Autodesk Inventor part; units mm, degrees
(part 3 of 4)
  arc A667 (-372.9607, 402.336) -> (-375.7104, 397.5735) centre (-372.9607, 399.161) ccw
  arc A668 (-368.5096, 385.1015) -> (-363.0104, 385.1015) centre (-365.76, 386.689) ccw
  line L673 (-355.8096, 397.5735) -> (-363.0104, 385.1015)
  line L674 (-372.9607, 402.336) -> (-358.5593, 402.336)
  arc A669 (-363.2031, 377.2287) -> (-368.7023, 377.2287) centre (-365.9527, 375.6412) ccw
  line L675 (-356.0023, 364.7567) -> (-363.2031, 377.2287)
  line L676 (-368.7023, 377.2287) -> (-375.9031, 364.7567)
  arc A670 (-375.9031, 364.7567) -> (-373.1534, 359.9942) centre (-373.1534, 363.1692) ccw
  line L677 (-373.1534, 359.9942) -> (-358.752, 359.9942)
  arc A671 (-358.752, 359.9942) -> (-356.0023, 364.7567) centre (-358.752, 363.1692) ccw
  line L678 (-314.1536, 58.9655) -> (-321.3544, 71.4375)
  arc A672 (-301.4536, 71.4375) -> (-304.2033, 76.2) centre (-304.2033, 73.025) ccw
  arc A673 (-318.6047, 76.2) -> (-321.3544, 71.4375) centre (-318.6047, 73.025) ccw
  arc A674 (-314.1536, 58.9655) -> (-308.6544, 58.9655) centre (-311.404, 60.553) ccw
  line L679 (-301.4536, 71.4375) -> (-308.6544, 58.9655)
  line L680 (-318.6047, 76.2) -> (-304.2033, 76.2)
  arc A675 (-308.8471, 51.0927) -> (-314.3463, 51.0927) centre (-311.5967, 49.5052) ccw
  line L681 (-301.6463, 38.6207) -> (-308.8471, 51.0927)
  line L682 (-314.3463, 51.0927) -> (-321.5471, 38.6207)
  arc A676 (-321.5471, 38.6207) -> (-318.7974, 33.8582) centre (-318.7974, 37.0332) ccw
  line L683 (-318.7974, 33.8582) -> (-304.396, 33.8582)
  arc A677 (-304.396, 33.8582) -> (-301.6463, 38.6207) centre (-304.396, 37.0332) ccw
  line L684 (-314.1536, 113.3215) -> (-321.3544, 125.7935)
  arc A678 (-301.4536, 125.7935) -> (-304.2033, 130.556) centre (-304.2033, 127.381) ccw
  arc A679 (-318.6047, 130.556) -> (-321.3544, 125.7935) centre (-318.6047, 127.381) ccw
  arc A680 (-314.1536, 113.3215) -> (-308.6544, 113.3215) centre (-311.404, 114.909) ccw
  line L685 (-301.4536, 125.7935) -> (-308.6544, 113.3215)
  line L686 (-318.6047, 130.556) -> (-304.2033, 130.556)
  arc A681 (-308.8471, 105.4487) -> (-314.3463, 105.4487) centre (-311.5967, 103.8612) ccw
  line L687 (-301.6463, 92.9767) -> (-308.8471, 105.4487)
  line L688 (-314.3463, 105.4487) -> (-321.5471, 92.9767)
  arc A682 (-321.5471, 92.9767) -> (-318.7974, 88.2142) centre (-318.7974, 91.3892) ccw
  line L689 (-318.7974, 88.2142) -> (-304.396, 88.2142)
  arc A683 (-304.396, 88.2142) -> (-301.6463, 92.9767) centre (-304.396, 91.3892) ccw
  line L690 (-314.1536, 167.6775) -> (-321.3544, 180.1495)
  arc A684 (-301.4536, 180.1495) -> (-304.2033, 184.912) centre (-304.2033, 181.737) ccw
  arc A685 (-318.6047, 184.912) -> (-321.3544, 180.1495) centre (-318.6047, 181.737) ccw
  arc A686 (-314.1536, 167.6775) -> (-308.6544, 167.6775) centre (-311.404, 169.265) ccw
  line L691 (-301.4536, 180.1495) -> (-308.6544, 167.6775)
  line L692 (-318.6047, 184.912) -> (-304.2033, 184.912)
  arc A687 (-308.8471, 159.8047) -> (-314.3463, 159.8047) centre (-311.5967, 158.2172) ccw
  line L693 (-301.6463, 147.3327) -> (-308.8471, 159.8047)
  line L694 (-314.3463, 159.8047) -> (-321.5471, 147.3327)
  arc A688 (-321.5471, 147.3327) -> (-318.7974, 142.5702) centre (-318.7974, 145.7452) ccw
  line L695 (-318.7974, 142.5702) -> (-304.396, 142.5702)
  arc A689 (-304.396, 142.5702) -> (-301.6463, 147.3327) centre (-304.396, 145.7452) ccw
  line L696 (-314.1536, 222.0335) -> (-321.3544, 234.5055)
  arc A690 (-301.4536, 234.5055) -> (-304.2033, 239.268) centre (-304.2033, 236.093) ccw
  arc A691 (-318.6047, 239.268) -> (-321.3544, 234.5055) centre (-318.6047, 236.093) ccw
  arc A692 (-314.1536, 222.0335) -> (-308.6544, 222.0335) centre (-311.404, 223.621) ccw
  line L697 (-301.4536, 234.5055) -> (-308.6544, 222.0335)
  line L698 (-318.6047, 239.268) -> (-304.2033, 239.268)
  arc A693 (-308.8471, 214.1607) -> (-314.3463, 214.1607) centre (-311.5967, 212.5732) ccw
  line L699 (-301.6463, 201.6887) -> (-308.8471, 214.1607)
  line L700 (-314.3463, 214.1607) -> (-321.5471, 201.6887)
  arc A694 (-321.5471, 201.6887) -> (-318.7974, 196.9262) centre (-318.7974, 200.1012) ccw
  line L701 (-318.7974, 196.9262) -> (-304.396, 196.9262)
  arc A695 (-304.396, 196.9262) -> (-301.6463, 201.6887) centre (-304.396, 200.1012) ccw
  line L702 (-314.1536, 276.3895) -> (-321.3544, 288.8615)
  arc A696 (-301.4536, 288.8615) -> (-304.2033, 293.624) centre (-304.2033, 290.449) ccw
  arc A697 (-318.6047, 293.624) -> (-321.3544, 288.8615) centre (-318.6047, 290.449) ccw
  arc A698 (-314.1536, 276.3895) -> (-308.6544, 276.3895) centre (-311.404, 277.977) ccw
  line L703 (-301.4536, 288.8615) -> (-308.6544, 276.3895)
  line L704 (-318.6047, 293.624) -> (-304.2033, 293.624)
  arc A699 (-308.8471, 268.5167) -> (-314.3463, 268.5167) centre (-311.5967, 266.9292) ccw
  line L705 (-301.6463, 256.0447) -> (-308.8471, 268.5167)
  line L706 (-314.3463, 268.5167) -> (-321.5471, 256.0447)
  arc A700 (-321.5471, 256.0447) -> (-318.7974, 251.2822) centre (-318.7974, 254.4572) ccw
  line L707 (-318.7974, 251.2822) -> (-304.396, 251.2822)
  arc A701 (-304.396, 251.2822) -> (-301.6463, 256.0447) centre (-304.396, 254.4572) ccw
  line L708 (-314.1536, 330.7455) -> (-321.3544, 343.2175)
  arc A702 (-301.4536, 343.2175) -> (-304.2033, 347.98) centre (-304.2033, 344.805) ccw
  arc A703 (-318.6047, 347.98) -> (-321.3544, 343.2175) centre (-318.6047, 344.805) ccw
  arc A704 (-314.1536, 330.7455) -> (-308.6544, 330.7455) centre (-311.404, 332.333) ccw
  line L709 (-301.4536, 343.2175) -> (-308.6544, 330.7455)
  line L710 (-318.6047, 347.98) -> (-304.2033, 347.98)
  arc A705 (-308.8471, 322.8727) -> (-314.3463, 322.8727) centre (-311.5967, 321.2852) ccw
  line L711 (-301.6463, 310.4007) -> (-308.8471, 322.8727)
  line L712 (-314.3463, 322.8727) -> (-321.5471, 310.4007)
  arc A706 (-321.5471, 310.4007) -> (-318.7974, 305.6382) centre (-318.7974, 308.8132) ccw
  line L713 (-318.7974, 305.6382) -> (-304.396, 305.6382)
  arc A707 (-304.396, 305.6382) -> (-301.6463, 310.4007) centre (-304.396, 308.8132) ccw
  line L714 (-314.1536, 385.1015) -> (-321.3544, 397.5735)
  arc A708 (-301.4536, 397.5735) -> (-304.2033, 402.336) centre (-304.2033, 399.161) ccw
  arc A709 (-318.6047, 402.336) -> (-321.3544, 397.5735) centre (-318.6047, 399.161) ccw
  arc A710 (-314.1536, 385.1015) -> (-308.6544, 385.1015) centre (-311.404, 386.689) ccw
  line L715 (-301.4536, 397.5735) -> (-308.6544, 385.1015)
  line L716 (-318.6047, 402.336) -> (-304.2033, 402.336)
  arc A711 (-308.8471, 377.2287) -> (-314.3463, 377.2287) centre (-311.5967, 375.6412) ccw
  line L717 (-301.6463, 364.7567) -> (-308.8471, 377.2287)
  line L718 (-314.3463, 377.2287) -> (-321.5471, 364.7567)
  arc A712 (-321.5471, 364.7567) -> (-318.7974, 359.9942) centre (-318.7974, 363.1692) ccw
  line L719 (-318.7974, 359.9942) -> (-304.396, 359.9942)
  arc A713 (-304.396, 359.9942) -> (-301.6463, 364.7567) centre (-304.396, 363.1692) ccw
  line L720 (-259.7976, 58.9655) -> (-266.9984, 71.4375)
  arc A714 (-247.0976, 71.4375) -> (-249.8473, 76.2) centre (-249.8473, 73.025) ccw
  arc A715 (-264.2487, 76.2) -> (-266.9984, 71.4375) centre (-264.2487, 73.025) ccw
  arc A716 (-259.7976, 58.9655) -> (-254.2984, 58.9655) centre (-257.048, 60.553) ccw
  line L721 (-247.0976, 71.4375) -> (-254.2984, 58.9655)
  line L722 (-264.2487, 76.2) -> (-249.8473, 76.2)
  arc A717 (-254.4911, 51.0927) -> (-259.9903, 51.0927) centre (-257.2407, 49.5052) ccw
  line L723 (-247.2903, 38.6207) -> (-254.4911, 51.0927)
  line L724 (-259.9903, 51.0927) -> (-267.1911, 38.6207)
  arc A718 (-267.1911, 38.6207) -> (-264.4414, 33.8582) centre (-264.4414, 37.0332) ccw
  line L725 (-264.4414, 33.8582) -> (-250.04, 33.8582)
  arc A719 (-250.04, 33.8582) -> (-247.2903, 38.6207) centre (-250.04, 37.0332) ccw
  line L726 (-259.7976, 113.3215) -> (-266.9984, 125.7935)
  arc A720 (-247.0976, 125.7935) -> (-249.8473, 130.556) centre (-249.8473, 127.381) ccw
  arc A721 (-264.2487, 130.556) -> (-266.9984, 125.7935) centre (-264.2487, 127.381) ccw
  arc A722 (-259.7976, 113.3215) -> (-254.2984, 113.3215) centre (-257.048, 114.909) ccw
  line L727 (-247.0976, 125.7935) -> (-254.2984, 113.3215)
  line L728 (-264.2487, 130.556) -> (-249.8473, 130.556)
  arc A723 (-254.4911, 105.4487) -> (-259.9903, 105.4487) centre (-257.2407, 103.8612) ccw
  line L729 (-247.2903, 92.9767) -> (-254.4911, 105.4487)
  line L730 (-259.9903, 105.4487) -> (-267.1911, 92.9767)
  arc A724 (-267.1911, 92.9767) -> (-264.4414, 88.2142) centre (-264.4414, 91.3892) ccw
  line L731 (-264.4414, 88.2142) -> (-250.04, 88.2142)
  arc A725 (-250.04, 88.2142) -> (-247.2903, 92.9767) centre (-250.04, 91.3892) ccw
  line L732 (-259.7976, 167.6775) -> (-266.9984, 180.1495)
  arc A726 (-247.0976, 180.1495) -> (-249.8473, 184.912) centre (-249.8473, 181.737) ccw
  arc A727 (-264.2487, 184.912) -> (-266.9984, 180.1495) centre (-264.2487, 181.737) ccw
  arc A728 (-259.7976, 167.6775) -> (-254.2984, 167.6775) centre (-257.048, 169.265) ccw
  line L733 (-247.0976, 180.1495) -> (-254.2984, 167.6775)
  line L734 (-264.2487, 184.912) -> (-249.8473, 184.912)
  arc A729 (-254.4911, 159.8047) -> (-259.9903, 159.8047) centre (-257.2407, 158.2172) ccw
  line L735 (-247.2903, 147.3327) -> (-254.4911, 159.8047)
  line L736 (-259.9903, 159.8047) -> (-267.1911, 147.3327)
  arc A730 (-267.1911, 147.3327) -> (-264.4414, 142.5702) centre (-264.4414, 145.7452) ccw
  line L737 (-264.4414, 142.5702) -> (-250.04, 142.5702)
  arc A731 (-250.04, 142.5702) -> (-247.2903, 147.3327) centre (-250.04, 145.7452) ccw
  line L738 (-259.7976, 222.0335) -> (-266.9984, 234.5055)
  arc A732 (-247.0976, 234.5055) -> (-249.8473, 239.268) centre (-249.8473, 236.093) ccw
  arc A733 (-264.2487, 239.268) -> (-266.9984, 234.5055) centre (-264.2487, 236.093) ccw
  arc A734 (-259.7976, 222.0335) -> (-254.2984, 222.0335) centre (-257.048, 223.621) ccw
  line L739 (-247.0976, 234.5055) -> (-254.2984, 222.0335)
  line L740 (-264.2487, 239.268) -> (-249.8473, 239.268)
  arc A735 (-254.4911, 214.1607) -> (-259.9903, 214.1607) centre (-257.2407, 212.5732) ccw
  line L741 (-247.2903, 201.6887) -> (-254.4911, 214.1607)
  line L742 (-259.9903, 214.1607) -> (-267.1911, 201.6887)
  arc A736 (-267.1911, 201.6887) -> (-264.4414, 196.9262) centre (-264.4414, 200.1012) ccw
  line L743 (-264.4414, 196.9262) -> (-250.04, 196.9262)
  arc A737 (-250.04, 196.9262) -> (-247.2903, 201.6887) centre (-250.04, 200.1012) ccw
  line L744 (-259.7976, 276.3895) -> (-266.9984, 288.8615)
  arc A738 (-247.0976, 288.8615) -> (-249.8473, 293.624) centre (-249.8473, 290.449) ccw
  arc A739 (-264.2487, 293.624) -> (-266.9984, 288.8615) centre (-264.2487, 290.449) ccw
  arc A740 (-259.7976, 276.3895) -> (-254.2984, 276.3895) centre (-257.048, 277.977) ccw
  line L745 (-247.0976, 288.8615) -> (-254.2984, 276.3895)
  line L746 (-264.2487, 293.624) -> (-249.8473, 293.624)
  arc A741 (-254.4911, 268.5167) -> (-259.9903, 268.5167) centre (-257.2407, 266.9292) ccw
  line L747 (-247.2903, 256.0447) -> (-254.4911, 268.5167)
  line L748 (-259.9903, 268.5167) -> (-267.1911, 256.0447)
  arc A742 (-267.1911, 256.0447) -> (-264.4414, 251.2822) centre (-264.4414, 254.4572) ccw
  line L749 (-264.4414, 251.2822) -> (-250.04, 251.2822)
  arc A743 (-250.04, 251.2822) -> (-247.2903, 256.0447) centre (-250.04, 254.4572) ccw
  line L750 (-259.7976, 330.7455) -> (-266.9984, 343.2175)
  arc A744 (-247.0976, 343.2175) -> (-249.8473, 347.98) centre (-249.8473, 344.805) ccw
  arc A745 (-264.2487, 347.98) -> (-266.9984, 343.2175) centre (-264.2487, 344.805) ccw
  arc A746 (-259.7976, 330.7455) -> (-254.2984, 330.7455) centre (-257.048, 332.333) ccw
  line L751 (-247.0976, 343.2175) -> (-254.2984, 330.7455)
  line L752 (-264.2487, 347.98) -> (-249.8473, 347.98)
  arc A747 (-254.4911, 322.8727) -> (-259.9903, 322.8727) centre (-257.2407, 321.2852) ccw
  line L753 (-247.2903, 310.4007) -> (-254.4911, 322.8727)
  line L754 (-259.9903, 322.8727) -> (-267.1911, 310.4007)
  arc A748 (-267.1911, 310.4007) -> (-264.4414, 305.6382) centre (-264.4414, 308.8132) ccw
  line L755 (-264.4414, 305.6382) -> (-250.04, 305.6382)
  arc A749 (-250.04, 305.6382) -> (-247.2903, 310.4007) centre (-250.04, 308.8132) ccw
  line L756 (-259.7976, 385.1015) -> (-266.9984, 397.5735)
  arc A750 (-247.0976, 397.5735) -> (-249.8473, 402.336) centre (-249.8473, 399.161) ccw
  arc A751 (-264.2487, 402.336) -> (-266.9984, 397.5735) centre (-264.2487, 399.161) ccw
  arc A752 (-259.7976, 385.1015) -> (-254.2984, 385.1015) centre (-257.048, 386.689) ccw
  line L757 (-247.0976, 397.5735) -> (-254.2984, 385.1015)
  line L758 (-264.2487, 402.336) -> (-249.8473, 402.336)
  arc A753 (-254.4911, 377.2287) -> (-259.9903, 377.2287) centre (-257.2407, 375.6412) ccw
  line L759 (-247.2903, 364.7567) -> (-254.4911, 377.2287)
  line L760 (-259.9903, 377.2287) -> (-267.1911, 364.7567)
  arc A754 (-267.1911, 364.7567) -> (-264.4414, 359.9942) centre (-264.4414, 363.1692) ccw
  line L761 (-264.4414, 359.9942) -> (-250.04, 359.9942)
  arc A755 (-250.04, 359.9942) -> (-247.2903, 364.7567) centre (-250.04, 363.1692) ccw
  line L762 (-205.4416, 58.9655) -> (-212.6424, 71.4375)
  arc A756 (-192.7416, 71.4375) -> (-195.4913, 76.2) centre (-195.4913, 73.025) ccw
  arc A757 (-209.8927, 76.2) -> (-212.6424, 71.4375) centre (-209.8927, 73.025) ccw
  arc A758 (-205.4416, 58.9655) -> (-199.9424, 58.9655) centre (-202.692, 60.553) ccw
  line L763 (-192.7416, 71.4375) -> (-199.9424, 58.9655)
  line L764 (-209.8927, 76.2) -> (-195.4913, 76.2)
  arc A759 (-200.1351, 51.0927) -> (-205.6343, 51.0927) centre (-202.8847, 49.5052) ccw
  line L765 (-192.9343, 38.6207) -> (-200.1351, 51.0927)
  line L766 (-205.6343, 51.0927) -> (-212.8351, 38.6207)
  arc A760 (-212.8351, 38.6207) -> (-210.0854, 33.8582) centre (-210.0854, 37.0332) ccw
  line L767 (-210.0854, 33.8582) -> (-195.684, 33.8582)
  arc A761 (-195.684, 33.8582) -> (-192.9343, 38.6207) centre (-195.684, 37.0332) ccw
  line L768 (-205.4416, 113.3215) -> (-212.6424, 125.7935)
  arc A762 (-192.7416, 125.7935) -> (-195.4913, 130.556) centre (-195.4913, 127.381) ccw
  arc A763 (-209.8927, 130.556) -> (-212.6424, 125.7935) centre (-209.8927, 127.381) ccw
  arc A764 (-205.4416, 113.3215) -> (-199.9424, 113.3215) centre (-202.692, 114.909) ccw
  line L769 (-192.7416, 125.7935) -> (-199.9424, 113.3215)
  line L770 (-209.8927, 130.556) -> (-195.4913, 130.556)
  arc A765 (-200.1351, 105.4487) -> (-205.6343, 105.4487) centre (-202.8847, 103.8612) ccw
  line L771 (-192.9343, 92.9767) -> (-200.1351, 105.4487)
  line L772 (-205.6343, 105.4487) -> (-212.8351, 92.9767)
  arc A766 (-212.8351, 92.9767) -> (-210.0854, 88.2142) centre (-210.0854, 91.3892) ccw
  line L773 (-210.0854, 88.2142) -> (-195.684, 88.2142)
  arc A767 (-195.684, 88.2142) -> (-192.9343, 92.9767) centre (-195.684, 91.3892) ccw
  line L774 (-205.4416, 167.6775) -> (-212.6424, 180.1495)
  arc A768 (-192.7416, 180.1495) -> (-195.4913, 184.912) centre (-195.4913, 181.737) ccw
  arc A769 (-209.8927, 184.912) -> (-212.6424, 180.1495) centre (-209.8927, 181.737) ccw
  arc A770 (-205.4416, 167.6775) -> (-199.9424, 167.6775) centre (-202.692, 169.265) ccw
  line L775 (-192.7416, 180.1495) -> (-199.9424, 167.6775)
  line L776 (-209.8927, 184.912) -> (-195.4913, 184.912)
  arc A771 (-200.1351, 159.8047) -> (-205.6343, 159.8047) centre (-202.8847, 158.2172) ccw
  line L777 (-192.9343, 147.3327) -> (-200.1351, 159.8047)
  line L778 (-205.6343, 159.8047) -> (-212.8351, 147.3327)
  arc A772 (-212.8351, 147.3327) -> (-210.0854, 142.5702) centre (-210.0854, 145.7452) ccw
  line L779 (-210.0854, 142.5702) -> (-195.684, 142.5702)
  arc A773 (-195.684, 142.5702) -> (-192.9343, 147.3327) centre (-195.684, 145.7452) ccw
  line L780 (-205.4416, 222.0335) -> (-212.6424, 234.5055)
  arc A774 (-192.7416, 234.5055) -> (-195.4913, 239.268) centre (-195.4913, 236.093) ccw
  arc A775 (-209.8927, 239.268) -> (-212.6424, 234.5055) centre (-209.8927, 236.093) ccw
  arc A776 (-205.4416, 222.0335) -> (-199.9424, 222.0335) centre (-202.692, 223.621) ccw
  line L781 (-192.7416, 234.5055) -> (-199.9424, 222.0335)
  line L782 (-209.8927, 239.268) -> (-195.4913, 239.268)
  arc A777 (-200.1351, 214.1607) -> (-205.6343, 214.1607) centre (-202.8847, 212.5732) ccw
  line L783 (-192.9343, 201.6887) -> (-200.1351, 214.1607)
  line L784 (-205.6343, 214.1607) -> (-212.8351, 201.6887)
  arc A778 (-212.8351, 201.6887) -> (-210.0854, 196.9262) centre (-210.0854, 200.1012) ccw
  line L785 (-210.0854, 196.9262) -> (-195.684, 196.9262)
  arc A779 (-195.684, 196.9262) -> (-192.9343, 201.6887) centre (-195.684, 200.1012) ccw
  line L786 (-205.4416, 276.3895) -> (-212.6424, 288.8615)
  arc A780 (-192.7416, 288.8615) -> (-195.4913, 293.624) centre (-195.4913, 290.449) ccw
  arc A781 (-209.8927, 293.624) -> (-212.6424, 288.8615) centre (-209.8927, 290.449) ccw
  arc A782 (-205.4416, 276.3895) -> (-199.9424, 276.3895) centre (-202.692, 277.977) ccw
  line L787 (-192.7416, 288.8615) -> (-199.9424, 276.3895)
  line L788 (-209.8927, 293.624) -> (-195.4913, 293.624)
  arc A783 (-200.1351, 268.5167) -> (-205.6343, 268.5167) centre (-202.8847, 266.9292) ccw
  line L789 (-192.9343, 256.0447) -> (-200.1351, 268.5167)
  line L790 (-205.6343, 268.5167) -> (-212.8351, 256.0447)
  arc A784 (-212.8351, 256.0447) -> (-210.0854, 251.2822) centre (-210.0854, 254.4572) ccw
  line L791 (-210.0854, 251.2822) -> (-195.684, 251.2822)
  arc A785 (-195.684, 251.2822) -> (-192.9343, 256.0447) centre (-195.684, 254.4572) ccw
  line L792 (-205.4416, 330.7455) -> (-212.6424, 343.2175)
  arc A786 (-192.7416, 343.2175) -> (-195.4913, 347.98) centre (-195.4913, 344.805) ccw
  arc A787 (-209.8927, 347.98) -> (-212.6424, 343.2175) centre (-209.8927, 344.805) ccw
  arc A788 (-205.4416, 330.7455) -> (-199.9424, 330.7455) centre (-202.692, 332.333) ccw
  line L793 (-192.7416, 343.2175) -> (-199.9424, 330.7455)
  line L794 (-209.8927, 347.98) -> (-195.4913, 347.98)
  arc A789 (-200.1351, 322.8727) -> (-205.6343, 322.8727) centre (-202.8847, 321.2852) ccw
  line L795 (-192.9343, 310.4007) -> (-200.1351, 322.8727)
  line L796 (-205.6343, 322.8727) -> (-212.8351, 310.4007)
  arc A790 (-212.8351, 310.4007) -> (-210.0854, 305.6382) centre (-210.0854, 308.8132) ccw
  line L797 (-210.0854, 305.6382) -> (-195.684, 305.6382)
  arc A791 (-195.684, 305.6382) -> (-192.9343, 310.4007) centre (-195.684, 308.8132) ccw
  line L798 (-205.4416, 385.1015) -> (-212.6424, 397.5735)
  arc A792 (-192.7416, 397.5735) -> (-195.4913, 402.336) centre (-195.4913, 399.161) ccw
  arc A793 (-209.8927, 402.336) -> (-212.6424, 397.5735) centre (-209.8927, 399.161) ccw
  arc A794 (-205.4416, 385.1015) -> (-199.9424, 385.1015) centre (-202.692, 386.689) ccw
  line L799 (-192.7416, 397.5735) -> (-199.9424, 385.1015)
  line L800 (-209.8927, 402.336) -> (-195.4913, 402.336)
  arc A795 (-200.1351, 377.2287) -> (-205.6343, 377.2287) centre (-202.8847, 375.6412) ccw
  line L801 (-192.9343, 364.7567) -> (-200.1351, 377.2287)
  line L802 (-205.6343, 377.2287) -> (-212.8351, 364.7567)
  arc A796 (-212.8351, 364.7567) -> (-210.0854, 359.9942) centre (-210.0854, 363.1692) ccw
  line L803 (-210.0854, 359.9942) -> (-195.684, 359.9942)
  arc A797 (-195.684, 359.9942) -> (-192.9343, 364.7567) centre (-195.684, 363.1692) ccw
  line L804 (-151.0856, 58.9655) -> (-158.2864, 71.4375)
  arc A798 (-138.3856, 71.4375) -> (-141.1353, 76.2) centre (-141.1353, 73.025) ccw
  arc A799 (-155.5367, 76.2) -> (-158.2864, 71.4375) centre (-155.5367, 73.025) ccw
  arc A800 (-151.0856, 58.9655) -> (-145.5864, 58.9655) centre (-148.336, 60.553) ccw
  line L805 (-138.3856, 71.4375) -> (-145.5864, 58.9655)
  line L806 (-155.5367, 76.2) -> (-141.1353, 76.2)
  arc A801 (-145.7791, 51.0927) -> (-151.2783, 51.0927) centre (-148.5287, 49.5052) ccw
  line L807 (-138.5783, 38.6207) -> (-145.7791, 51.0927)
  line L808 (-151.2783, 51.0927) -> (-158.4791, 38.6207)
  arc A802 (-158.4791, 38.6207) -> (-155.7294, 33.8582) centre (-155.7294, 37.0332) ccw
  line L809 (-155.7294, 33.8582) -> (-141.328, 33.8582)
  arc A803 (-141.328, 33.8582) -> (-138.5783, 38.6207) centre (-141.328, 37.0332) ccw
  line L810 (-151.0856, 113.3215) -> (-158.2864, 125.7935)
  arc A804 (-138.3856, 125.7935) -> (-141.1353, 130.556) centre (-141.1353, 127.381) ccw
  arc A805 (-155.5367, 130.556) -> (-158.2864, 125.7935) centre (-155.5367, 127.381) ccw
  arc A806 (-151.0856, 113.3215) -> (-145.5864, 113.3215) centre (-148.336, 114.909) ccw
  line L811 (-138.3856, 125.7935) -> (-145.5864, 113.3215)
  line L812 (-155.5367, 130.556) -> (-141.1353, 130.556)
  arc A807 (-145.7791, 105.4487) -> (-151.2783, 105.4487) centre (-148.5287, 103.8612) ccw
  line L813 (-138.5783, 92.9767) -> (-145.7791, 105.4487)
  line L814 (-151.2783, 105.4487) -> (-158.4791, 92.9767)
  arc A808 (-158.4791, 92.9767) -> (-155.7294, 88.2142) centre (-155.7294, 91.3892) ccw
  line L815 (-155.7294, 88.2142) -> (-141.328, 88.2142)
  arc A809 (-141.328, 88.2142) -> (-138.5783, 92.9767) centre (-141.328, 91.3892) ccw
  line L816 (-151.0856, 167.6775) -> (-158.2864, 180.1495)
  arc A810 (-138.3856, 180.1495) -> (-141.1353, 184.912) centre (-141.1353, 181.737) ccw
  arc A811 (-155.5367, 184.912) -> (-158.2864, 180.1495) centre (-155.5367, 181.737) ccw
  arc A812 (-151.0856, 167.6775) -> (-145.5864, 167.6775) centre (-148.336, 169.265) ccw
  line L817 (-138.3856, 180.1495) -> (-145.5864, 167.6775)
  line L818 (-155.5367, 184.912) -> (-141.1353, 184.912)
  arc A813 (-145.7791, 159.8047) -> (-151.2783, 159.8047) centre (-148.5287, 158.2172) ccw
  line L819 (-138.5783, 147.3327) -> (-145.7791, 159.8047)
  line L820 (-151.2783, 159.8047) -> (-158.4791, 147.3327)
  arc A814 (-158.4791, 147.3327) -> (-155.7294, 142.5702) centre (-155.7294, 145.7452) ccw
  line L821 (-155.7294, 142.5702) -> (-141.328, 142.5702)
  arc A815 (-141.328, 142.5702) -> (-138.5783, 147.3327) centre (-141.328, 145.7452) ccw
  line L822 (-151.0856, 222.0335) -> (-158.2864, 234.5055)
  arc A816 (-138.3856, 234.5055) -> (-141.1353, 239.268) centre (-141.1353, 236.093) ccw
  arc A817 (-155.5367, 239.268) -> (-158.2864, 234.5055) centre (-155.5367, 236.093) ccw
  arc A818 (-151.0856, 222.0335) -> (-145.5864, 222.0335) centre (-148.336, 223.621) ccw
  line L823 (-138.3856, 234.5055) -> (-145.5864, 222.0335)
  line L824 (-155.5367, 239.268) -> (-141.1353, 239.268)
  arc A819 (-145.7791, 214.1607) -> (-151.2783, 214.1607) centre (-148.5287, 212.5732) ccw
  line L825 (-138.5783, 201.6887) -> (-145.7791, 214.1607)
  line L826 (-151.2783, 214.1607) -> (-158.4791, 201.6887)
  arc A820 (-158.4791, 201.6887) -> (-155.7294, 196.9262) centre (-155.7294, 200.1012) ccw
  line L827 (-155.7294, 196.9262) -> (-141.328, 196.9262)
  arc A821 (-141.328, 196.9262) -> (-138.5783, 201.6887) centre (-141.328, 200.1012) ccw
  line L828 (-151.0856, 276.3895) -> (-158.2864, 288.8615)
  arc A822 (-138.3856, 288.8615) -> (-141.1353, 293.624) centre (-141.1353, 290.449) ccw
  arc A823 (-155.5367, 293.624) -> (-158.2864, 288.8615) centre (-155.5367, 290.449) ccw
  arc A824 (-151.0856, 276.3895) -> (-145.5864, 276.3895) centre (-148.336, 277.977) ccw
  line L829 (-138.3856, 288.8615) -> (-145.5864, 276.3895)
  line L830 (-155.5367, 293.624) -> (-141.1353, 293.624)
  arc A825 (-145.7791, 268.5167) -> (-151.2783, 268.5167) centre (-148.5287, 266.9292) ccw
  line L831 (-138.5783, 256.0447) -> (-145.7791, 268.5167)
  line L832 (-151.2783, 268.5167) -> (-158.4791, 256.0447)
  arc A826 (-158.4791, 256.0447) -> (-155.7294, 251.2822) centre (-155.7294, 254.4572) ccw
  line L833 (-155.7294, 251.2822) -> (-141.328, 251.2822)
  arc A827 (-141.328, 251.2822) -> (-138.5783, 256.0447) centre (-141.328, 254.4572) ccw
  line L834 (-151.0856, 330.7455) -> (-158.2864, 343.2175)
  arc A828 (-138.3856, 343.2175) -> (-141.1353, 347.98) centre (-141.1353, 344.805) ccw
  arc A829 (-155.5367, 347.98) -> (-158.2864, 343.2175) centre (-155.5367, 344.805) ccw
  arc A830 (-151.0856, 330.7455) -> (-145.5864, 330.7455) centre (-148.336, 332.333) ccw
  line L835 (-138.3856, 343.2175) -> (-145.5864, 330.7455)
  line L836 (-155.5367, 347.98) -> (-141.1353, 347.98)
  arc A831 (-145.7791, 322.8727) -> (-151.2783, 322.8727) centre (-148.5287, 321.2852) ccw
  line L837 (-138.5783, 310.4007) -> (-145.7791, 322.8727)
  line L838 (-151.2783, 322.8727) -> (-158.4791, 310.4007)
  arc A832 (-158.4791, 310.4007) -> (-155.7294, 305.6382) centre (-155.7294, 308.8132) ccw
  line L839 (-155.7294, 305.6382) -> (-141.328, 305.6382)
  arc A833 (-141.328, 305.6382) -> (-138.5783, 310.4007) centre (-141.328, 308.8132) ccw
  line L840 (-151.0856, 385.1015) -> (-158.2864, 397.5735)
  arc A834 (-138.3856, 397.5735) -> (-141.1353, 402.336) centre (-141.1353, 399.161) ccw
  arc A835 (-155.5367, 402.336) -> (-158.2864, 397.5735) centre (-155.5367, 399.161) ccw
  arc A836 (-151.0856, 385.1015) -> (-145.5864, 385.1015) centre (-148.336, 386.689) ccw
  line L841 (-138.3856, 397.5735) -> (-145.5864, 385.1015)
  line L842 (-155.5367, 402.336) -> (-141.1353, 402.336)
  arc A837 (-145.7791, 377.2287) -> (-151.2783, 377.2287) centre (-148.5287, 375.6412) ccw
  line L843 (-138.5783, 364.7567) -> (-145.7791, 377.2287)
  line L844 (-151.2783, 377.2287) -> (-158.4791, 364.7567)
  arc A838 (-158.4791, 364.7567) -> (-155.7294, 359.9942) centre (-155.7294, 363.1692) ccw
  line L845 (-155.7294, 359.9942) -> (-141.328, 359.9942)
  arc A839 (-141.328, 359.9942) -> (-138.5783, 364.7567) centre (-141.328, 363.1692) ccw
  line L846 (-96.7296, 58.9655) -> (-103.9304, 71.4375)
  arc A840 (-84.0296, 71.4375) -> (-86.7793, 76.2) centre (-86.7793, 73.025) ccw
  arc A841 (-101.1807, 76.2) -> (-103.9304, 71.4375) centre (-101.1807, 73.025) ccw
  arc A842 (-96.7296, 58.9655) -> (-91.2304, 58.9655) centre (-93.98, 60.553) ccw
  line L847 (-84.0296, 71.4375) -> (-91.2304, 58.9655)
  line L848 (-101.1807, 76.2) -> (-86.7793, 76.2)
  arc A843 (-91.4231, 51.0927) -> (-96.9223, 51.0927) centre (-94.1727, 49.5052) ccw
  line L849 (-84.2223, 38.6207) -> (-91.4231, 51.0927)
  line L850 (-96.9223, 51.0927) -> (-104.1231, 38.6207)
  arc A844 (-104.1231, 38.6207) -> (-101.3734, 33.8582) centre (-101.3734, 37.0332) ccw
  line L851 (-101.3734, 33.8582) -> (-86.972, 33.8582)
  arc A845 (-86.972, 33.8582) -> (-84.2223, 38.6207) centre (-86.972, 37.0332) ccw
  line L852 (-96.7296, 113.3215) -> (-103.9304, 125.7935)
  arc A846 (-84.0296, 125.7935) -> (-86.7793, 130.556) centre (-86.7793, 127.381) ccw
  arc A847 (-101.1807, 130.556) -> (-103.9304, 125.7935) centre (-101.1807, 127.381) ccw
  arc A848 (-96.7296, 113.3215) -> (-91.2304, 113.3215) centre (-93.98, 114.909) ccw
  line L853 (-84.0296, 125.7935) -> (-91.2304, 113.3215)
  line L854 (-101.1807, 130.556) -> (-86.7793, 130.556)
  arc A849 (-91.4231, 105.4487) -> (-96.9223, 105.4487) centre (-94.1727, 103.8612) ccw
  line L855 (-84.2223, 92.9767) -> (-91.4231, 105.4487)
  line L856 (-96.9223, 105.4487) -> (-104.1231, 92.9767)
  arc A850 (-104.1231, 92.9767) -> (-101.3734, 88.2142) centre (-101.3734, 91.3892) ccw
  line L857 (-101.3734, 88.2142) -> (-86.972, 88.2142)
  arc A851 (-86.972, 88.2142) -> (-84.2223, 92.9767) centre (-86.972, 91.3892) ccw
  line L858 (-96.7296, 167.6775) -> (-103.9304, 180.1495)
  arc A852 (-84.0296, 180.1495) -> (-86.7793, 184.912) centre (-86.7793, 181.737) ccw
  arc A853 (-101.1807, 184.912) -> (-103.9304, 180.1495) centre (-101.1807, 181.737) ccw
  arc A854 (-96.7296, 167.6775) -> (-91.2304, 167.6775) centre (-93.98, 169.265) ccw
  line L859 (-84.0296, 180.1495) -> (-91.2304, 167.6775)
  line L860 (-101.1807, 184.912) -> (-86.7793, 184.912)
  arc A855 (-91.4231, 159.8047) -> (-96.9223, 159.8047) centre (-94.1727, 158.2172) ccw
  line L861 (-84.2223, 147.3327) -> (-91.4231, 159.8047)
  line L862 (-96.9223, 159.8047) -> (-104.1231, 147.3327)
  arc A856 (-104.1231, 147.3327) -> (-101.3734, 142.5702) centre (-101.3734, 145.7452) ccw
  line L863 (-101.3734, 142.5702) -> (-86.972, 142.5702)
  arc A857 (-86.972, 142.5702) -> (-84.2223, 147.3327) centre (-86.972, 145.7452) ccw
  line L864 (-96.7296, 222.0335) -> (-103.9304, 234.5055)
  arc A858 (-84.0296, 234.5055) -> (-86.7793, 239.268) centre (-86.7793, 236.093) ccw
  arc A859 (-101.1807, 239.268) -> (-103.9304, 234.5055) centre (-101.1807, 236.093) ccw
  arc A860 (-96.7296, 222.0335) -> (-91.2304, 222.0335) centre (-93.98, 223.621) ccw
  line L865 (-84.0296, 234.5055) -> (-91.2304, 222.0335)
  line L866 (-101.1807, 239.268) -> (-86.7793, 239.268)
  arc A861 (-91.4231, 214.1607) -> (-96.9223, 214.1607) centre (-94.1727, 212.5732) ccw
  line L867 (-84.2223, 201.6887) -> (-91.4231, 214.1607)
  line L868 (-96.9223, 214.1607) -> (-104.1231, 201.6887)
  arc A862 (-104.1231, 201.6887) -> (-101.3734, 196.9262) centre (-101.3734, 200.1012) ccw
  line L869 (-101.3734, 196.9262) -> (-86.972, 196.9262)
  arc A863 (-86.972, 196.9262) -> (-84.2223, 201.6887) centre (-86.972, 200.1012) ccw
  line L870 (-96.7296, 276.3895) -> (-103.9304, 288.8615)
  arc A864 (-84.0296, 288.8615) -> (-86.7793, 293.624) centre (-86.7793, 290.449) ccw
  arc A865 (-101.1807, 293.624) -> (-103.9304, 288.8615) centre (-101.1807, 290.449) ccw
  arc A866 (-96.7296, 276.3895) -> (-91.2304, 276.3895) centre (-93.98, 277.977) ccw
  line L871 (-84.0296, 288.8615) -> (-91.2304, 276.3895)
  line L872 (-101.1807, 293.624) -> (-86.7793, 293.624)
  arc A867 (-91.4231, 268.5167) -> (-96.9223, 268.5167) centre (-94.1727, 266.9292) ccw
  line L873 (-84.2223, 256.0447) -> (-91.4231, 268.5167)
  line L874 (-96.9223, 268.5167) -> (-104.1231, 256.0447)
  arc A868 (-104.1231, 256.0447) -> (-101.3734, 251.2822) centre (-101.3734, 254.4572) ccw
  line L875 (-101.3734, 251.2822) -> (-86.972, 251.2822)
  arc A869 (-86.972, 251.2822) -> (-84.2223, 256.0447) centre (-86.972, 254.4572) ccw
  line L876 (-96.7296, 330.7455) -> (-103.9304, 343.2175)
  arc A870 (-84.0296, 343.2175) -> (-86.7793, 347.98) centre (-86.7793, 344.805) ccw
  arc A871 (-101.1807, 347.98) -> (-103.9304, 343.2175) centre (-101.1807, 344.805) ccw
  arc A872 (-96.7296, 330.7455) -> (-91.2304, 330.7455) centre (-93.98, 332.333) ccw
  line L877 (-84.0296, 343.2175) -> (-91.2304, 330.7455)
  line L878 (-101.1807, 347.98) -> (-86.7793, 347.98)
  arc A873 (-91.4231, 322.8727) -> (-96.9223, 322.8727) centre (-94.1727, 321.2852) ccw
  line L879 (-84.2223, 310.4007) -> (-91.4231, 322.8727)
  line L880 (-96.9223, 322.8727) -> (-104.1231, 310.4007)
  arc A874 (-104.1231, 310.4007) -> (-101.3734, 305.6382) centre (-101.3734, 308.8132) ccw
  line L881 (-101.3734, 305.6382) -> (-86.972, 305.6382)
  arc A875 (-86.972, 305.6382) -> (-84.2223, 310.4007) centre (-86.972, 308.8132) ccw
  line L882 (-96.7296, 385.1015) -> (-103.9304, 397.5735)
  arc A876 (-84.0296, 397.5735) -> (-86.7793, 402.336) centre (-86.7793, 399.161) ccw
  arc A877 (-101.1807, 402.336) -> (-103.9304, 397.5735) centre (-101.1807, 399.161) ccw
  arc A878 (-96.7296, 385.1015) -> (-91.2304, 385.1015) centre (-93.98, 386.689) ccw
  line L883 (-84.0296, 397.5735) -> (-91.2304, 385.1015)
  line L884 (-101.1807, 402.336) -> (-86.7793, 402.336)
  arc A879 (-91.4231, 377.2287) -> (-96.9223, 377.2287) centre (-94.1727, 375.6412) ccw
  line L885 (-84.2223, 364.7567) -> (-91.4231, 377.2287)
  line L886 (-96.9223, 377.2287) -> (-104.1231, 364.7567)
  arc A880 (-104.1231, 364.7567) -> (-101.3734, 359.9942) centre (-101.3734, 363.1692) ccw
  line L887 (-101.3734, 359.9942) -> (-86.972, 359.9942)
  arc A881 (-86.972, 359.9942) -> (-84.2223, 364.7567) centre (-86.972, 363.1692) ccw
  line L888 (-42.3736, 58.9655) -> (-49.5744, 71.4375)
  arc A882 (-29.6736, 71.4375) -> (-32.4233, 76.2) centre (-32.4233, 73.025) ccw
  arc A883 (-46.8247, 76.2) -> (-49.5744, 71.4375) centre (-46.8247, 73.025) ccw
  arc A884 (-42.3736, 58.9655) -> (-36.8744, 58.9655) centre (-39.624, 60.553) ccw
  line L889 (-29.6736, 71.4375) -> (-36.8744, 58.9655)
  line L890 (-46.8247, 76.2) -> (-32.4233, 76.2)
  arc A885 (-37.0671, 51.0927) -> (-42.5663, 51.0927) centre (-39.8167, 49.5052) ccw
  line L891 (-29.8663, 38.6207) -> (-37.0671, 51.0927)
  line L892 (-42.5663, 51.0927) -> (-49.7671, 38.6207)
  arc A886 (-49.7671, 38.6207) -> (-47.0174, 33.8582) centre (-47.0174, 37.0332) ccw
  line L893 (-47.0174, 33.8582) -> (-32.616, 33.8582)
  arc A887 (-32.616, 33.8582) -> (-29.8663, 38.6207) centre (-32.616, 37.0332) ccw
  line L894 (-42.3736, 113.3215) -> (-49.5744, 125.7935)
  arc A888 (-29.6736, 125.7935) -> (-32.4233, 130.556) centre (-32.4233, 127.381) ccw
  arc A889 (-46.8247, 130.556) -> (-49.5744, 125.7935) centre (-46.8247, 127.381) ccw
  arc A890 (-42.3736, 113.3215) -> (-36.8744, 113.3215) centre (-39.624, 114.909) ccw
  line L895 (-29.6736, 125.7935) -> (-36.8744, 113.3215)
  line L896 (-46.8247, 130.556) -> (-32.4233, 130.556)
  arc A891 (-37.0671, 105.4487) -> (-42.5663, 105.4487) centre (-39.8167, 103.8612) ccw
  line L897 (-29.8663, 92.9767) -> (-37.0671, 105.4487)
  line L898 (-42.5663, 105.4487) -> (-49.7671, 92.9767)
  arc A892 (-49.7671, 92.9767) -> (-47.0174, 88.2142) centre (-47.0174, 91.3892) ccw
  line L899 (-47.0174, 88.2142) -> (-32.616, 88.2142)
  arc A893 (-32.616, 88.2142) -> (-29.8663, 92.9767) centre (-32.616, 91.3892) ccw
  line L900 (-42.3736, 167.6775) -> (-49.5744, 180.1495)
  arc A894 (-29.6736, 180.1495) -> (-32.4233, 184.912) centre (-32.4233, 181.737) ccw
  arc A895 (-46.8247, 184.912) -> (-49.5744, 180.1495) centre (-46.8247, 181.737) ccw
  arc A896 (-42.3736, 167.6775) -> (-36.8744, 167.6775) centre (-39.624, 169.265) ccw
  line L901 (-29.6736, 180.1495) -> (-36.8744, 167.6775)
  line L902 (-46.8247, 184.912) -> (-32.4233, 184.912)
  arc A897 (-37.0671, 159.8047) -> (-42.5663, 159.8047) centre (-39.8167, 158.2172) ccw
  line L903 (-29.8663, 147.3327) -> (-37.0671, 159.8047)
  line L904 (-42.5663, 159.8047) -> (-49.7671, 147.3327)
  arc A898 (-49.7671, 147.3327) -> (-47.0174, 142.5702) centre (-47.0174, 145.7452) ccw
  line L905 (-47.0174, 142.5702) -> (-32.616, 142.5702)
  arc A899 (-32.616, 142.5702) -> (-29.8663, 147.3327) centre (-32.616, 145.7452) ccw
  line L906 (-42.3736, 222.0335) -> (-49.5744, 234.5055)
  arc A900 (-29.6736, 234.5055) -> (-32.4233, 239.268) centre (-32.4233, 236.093) ccw
  arc A901 (-46.8247, 239.268) -> (-49.5744, 234.5055) centre (-46.8247, 236.093) ccw
  arc A902 (-42.3736, 222.0335) -> (-36.8744, 222.0335) centre (-39.624, 223.621) ccw
  line L907 (-29.6736, 234.5055) -> (-36.8744, 222.0335)
  line L908 (-46.8247, 239.268) -> (-32.4233, 239.268)
  arc A903 (-37.0671, 214.1607) -> (-42.5663, 214.1607) centre (-39.8167, 212.5732) ccw
  line L909 (-29.8663, 201.6887) -> (-37.0671, 214.1607)
  line L910 (-42.5663, 214.1607) -> (-49.7671, 201.6887)
  arc A904 (-49.7671, 201.6887) -> (-47.0174, 196.9262) centre (-47.0174, 200.1012) ccw
  line L911 (-47.0174, 196.9262) -> (-32.616, 196.9262)
  arc A905 (-32.616, 196.9262) -> (-29.8663, 201.6887) centre (-32.616, 200.1012) ccw
  line L912 (-42.3736, 276.3895) -> (-49.5744, 288.8615)
  arc A906 (-29.6736, 288.8615) -> (-32.4233, 293.624) centre (-32.4233, 290.449) ccw
  arc A907 (-46.8247, 293.624) -> (-49.5744, 288.8615) centre (-46.8247, 290.449) ccw
  arc A908 (-42.3736, 276.3895) -> (-36.8744, 276.3895) centre (-39.624, 277.977) ccw
  line L913 (-29.6736, 288.8615) -> (-36.8744, 276.3895)
  line L914 (-46.8247, 293.624) -> (-32.4233, 293.624)
  arc A909 (-37.0671, 268.5167) -> (-42.5663, 268.5167) centre (-39.8167, 266.9292) ccw
  line L915 (-29.8663, 256.0447) -> (-37.0671, 268.5167)
  line L916 (-42.5663, 268.5167) -> (-49.7671, 256.0447)
  arc A910 (-49.7671, 256.0447) -> (-47.0174, 251.2822) centre (-47.0174, 254.4572) ccw
  line L917 (-47.0174, 251.2822) -> (-32.616, 251.2822)
  arc A911 (-32.616, 251.2822) -> (-29.8663, 256.0447) centre (-32.616, 254.4572) ccw
  line L918 (-42.3736, 330.7455) -> (-49.5744, 343.2175)
  arc A912 (-29.6736, 343.2175) -> (-32.4233, 347.98) centre (-32.4233, 344.805) ccw
  arc A913 (-46.8247, 347.98) -> (-49.5744, 343.2175) centre (-46.8247, 344.805) ccw
  arc A914 (-42.3736, 330.7455) -> (-36.8744, 330.7455) centre (-39.624, 332.333) ccw
  line L919 (-29.6736, 343.2175) -> (-36.8744, 330.7455)
  line L920 (-46.8247, 347.98) -> (-32.4233, 347.98)
  arc A915 (-37.0671, 322.8727) -> (-42.5663, 322.8727) centre (-39.8167, 321.2852) ccw
  line L921 (-29.8663, 310.4007) -> (-37.0671, 322.8727)
  line L922 (-42.5663, 322.8727) -> (-49.7671, 310.4007)
  arc A916 (-49.7671, 310.4007) -> (-47.0174, 305.6382) centre (-47.0174, 308.8132) ccw
  line L923 (-47.0174, 305.6382) -> (-32.616, 305.6382)
  arc A917 (-32.616, 305.6382) -> (-29.8663, 310.4007) centre (-32.616, 308.8132) ccw
  line L924 (-42.3736, 385.1015) -> (-49.5744, 397.5735)
  arc A918 (-29.6736, 397.5735) -> (-32.4233, 402.336) centre (-32.4233, 399.161) ccw
  arc A919 (-46.8247, 402.336) -> (-49.5744, 397.5735) centre (-46.8247, 399.161) ccw
  arc A920 (-42.3736, 385.1015) -> (-36.8744, 385.1015) centre (-39.624, 386.689) ccw
  line L925 (-29.6736, 397.5735) -> (-36.8744, 385.1015)
  line L926 (-46.8247, 402.336) -> (-32.4233, 402.336)
  arc A921 (-37.0671, 377.2287) -> (-42.5663, 377.2287) centre (-39.8167, 375.6412) ccw
  line L927 (-29.8663, 364.7567) -> (-37.0671, 377.2287)
  line L928 (-42.5663, 377.2287) -> (-49.7671, 364.7567)
  arc A922 (-49.7671, 364.7567) -> (-47.0174, 359.9942) centre (-47.0174, 363.1692) ccw
  line L929 (-47.0174, 359.9942) -> (-32.616, 359.9942)
  arc A923 (-32.616, 359.9942) -> (-29.8663, 364.7567) centre (-32.616, 363.1692) ccw
  point P0 (-1193.8, 79.756)
  point P1 (-1193.8, 134.112)
  point P2 (-1193.8, 188.468)
  point P3 (-1193.8, 242.824)
  point P4 (-1193.8, 297.18)
  point P5 (-1193.8, 351.536)
  point P6 (-1139.444, 25.4)
  point P7 (-1139.444, 79.756)
  point P8 (-1139.444, 134.112)
  point P9 (-1139.444, 188.468)
  point P10 (-1139.444, 242.824)
  point P11 (-1139.444, 297.18)
  point P12 (-1139.444, 351.536)
  point P13 (-1085.088, 25.4)
  point P14 (-1085.088, 79.756)
  point P15 (-1085.088, 134.112)
  point P16 (-1085.088, 188.468)
  point P17 (-1085.088, 242.824)
  point P18 (-1085.088, 297.18)
  point P19 (-1085.088, 351.536)
  point P20 (-1030.732, 25.4)
  point P21 (-1030.732, 79.756)
  point P22 (-1030.732, 134.112)
  point P23 (-1030.732, 188.468)
  point P24 (-1030.732, 242.824)
  point P25 (-1030.732, 297.18)
  point P26 (-1030.732, 351.536)
  point P27 (-976.376, 25.4)
  point P28 (-976.376, 79.756)
  point P29 (-976.376, 134.112)
  point P30 (-976.376, 188.468)
  point P31 (-976.376, 242.824)
  point P32 (-976.376, 297.18)
  point P33 (-976.376, 351.536)
  point P34 (-922.02, 25.4)
  point P35 (-922.02, 79.756)
  point P36 (-922.02, 134.112)
  point P37 (-922.02, 188.468)
  point P38 (-922.02, 242.824)
  point P39 (-922.02, 297.18)
  point P40 (-922.02, 351.536)
  point P41 (-867.664, 25.4)
  point P42 (-867.664, 79.756)
  point P43 (-867.664, 134.112)
  point P44 (-867.664, 188.468)
  point P45 (-867.664, 242.824)
  point P46 (-867.664, 297.18)
  point P47 (-867.664, 351.536)
  point P48 (-813.308, 25.4)
  point P49 (-813.308, 79.756)
  point P50 (-813.308, 134.112)
  point P51 (-813.308, 188.468)
  point P52 (-813.308, 242.824)
  point P53 (-813.308, 297.18)
  point P54 (-813.308, 351.536)
  point P55 (-758.952, 25.4)
  point P56 (-758.952, 79.756)
  point P57 (-758.952, 134.112)
  point P58 (-758.952, 188.468)
  point P59 (-758.952, 242.824)
  point P60 (-758.952, 297.18)
  point P61 (-758.952, 351.536)
  point P62 (-704.596, 25.4)
  point P63 (-704.596, 79.756)
  point P64 (-704.596, 134.112)
  point P65 (-704.596, 188.468)
  point P66 (-704.596, 242.824)
  point P67 (-704.596, 297.18)
  point P68 (-704.596, 351.536)
  point P69 (-650.24, 25.4)
  point P70 (-650.24, 79.756)
  point P71 (-650.24, 134.112)
  point P72 (-650.24, 188.468)
  point P73 (-650.24, 242.824)
  point P74 (-650.24, 297.18)
  point P75 (-650.24, 351.536)
  point P76 (-595.884, 25.4)
  point P77 (-595.884, 79.756)
  point P78 (-595.884, 134.112)
  point P79 (-595.884, 188.468)
  point P80 (-595.884, 242.824)
  point P81 (-595.884, 297.18)
  point P82 (-595.884, 351.536)
  point P83 (-541.528, 25.4)
  point P84 (-541.528, 79.756)
  point P85 (-541.528, 134.112)
  point P86 (-541.528, 188.468)
  point P87 (-541.528, 242.824)
  point P88 (-541.528, 297.18)
  point P89 (-541.528, 351.536)
  point P90 (-487.172, 25.4)
  point P91 (-487.172, 79.756)
  point P92 (-487.172, 134.112)
  point P93 (-487.172, 188.468)
  point P94 (-487.172, 242.824)
  point P95 (-487.172, 297.18)
  point P96 (-487.172, 351.536)
  point P97 (-432.816, 25.4)
  point P98 (-432.816, 79.756)
  point P99 (-432.816, 134.112)
  point P100 (-432.816, 188.468)
  point P101 (-432.816, 242.824)
  point P102 (-432.816, 297.18)
  point P103 (-432.816, 351.536)
  point P104 (-378.46, 25.4)
  point P105 (-378.46, 79.756)
  point P106 (-378.46, 134.112)
  point P107 (-378.46, 188.468)
  point P108 (-378.46, 242.824)
  point P109 (-378.46, 297.18)
  point P110 (-378.46, 351.536)
  point P111 (-324.104, 25.4)
  point P112 (-324.104, 79.756)
  point P113 (-324.104, 134.112)
  point P114 (-324.104, 188.468)
  point P115 (-324.104, 242.824)
  point P116 (-324.104, 297.18)
  point P117 (-324.104, 351.536)
  point P118 (-269.748, 25.4)
  point P119 (-269.748, 79.756)
  point P120 (-269.748, 134.112)
  point P121 (-269.748, 188.468)
  point P122 (-269.748, 242.824)
  point P123 (-269.748, 297.18)
  point P124 (-269.748, 351.536)
  point P125 (-215.392, 25.4)
  point P126 (-215.392, 79.756)
  point P127 (-215.392, 134.112)
  point P128 (-215.392, 188.468)
  point P129 (-215.392, 242.824)
  point P130 (-215.392, 297.18)
  point P131 (-215.392, 351.536)
  point P132 (-161.036, 25.4)
  point P133 (-161.036, 79.756)
  point P134 (-161.036, 134.112)
  point P135 (-161.036, 188.468)
  point P136 (-161.036, 242.824)
  point P137 (-161.036, 297.18)
  point P138 (-161.036, 351.536)
  point P139 (-106.68, 25.4)
  point P140 (-106.68, 79.756)
  point P141 (-106.68, 134.112)
  point P142 (-106.68, 188.468)
  point P143 (-106.68, 242.824)
  point P144 (-106.68, 297.18)
  point P145 (-106.68, 351.536)
  point P146 (-52.324, 25.4)
  point P147 (-52.324, 79.756)
  point P148 (-52.324, 134.112)
  point P149 (-52.324, 188.468)
  point P150 (-52.324, 242.824)
  point P151 (-52.324, 297.18)
  point P152 (-52.324, 351.536)
  dimension "d22" = 54.356
  dimension "d25" = 54.356
  constraints: 1852 end point, 1848 point on circle, 924 centre point, 5 tangent, 2 equal radius, 1 horizontal, 1 vertical, 4743 other
  measures "d22" distance of L4.end point (-1193.8, 79.756)
  measures "d25" distance of L4.end point (-1139.444, 25.4)